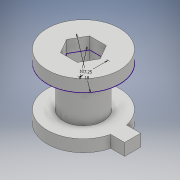
# Autodesk Inventor part: movingSpindle
Saved by Autodesk Inventor 2018 (Build 220112000, 112)
## iProperties
Created: 2018-11-25
Part Number: movingSpindle
Material: Generic
Document SubType Name: Modeling
Designer: Prakash
Density: 1 g/cm^3
Appearance: Default
Author: Prakash
Autodesk Inventor part; units mm, degrees
ref_plane "YZ Plane" through (0, 0, 0) normal (1, 0, 0) x (0, 1, 0)
ref_plane "XZ Plane" through (0, 0, 0) normal (0, 1, 0) x (-1, 0, 0)
ref_plane "XY Plane" through (0, 0, 0) normal (0, 0, 1) x (1, 0, 0)
sketch "Sketch1" plane through (0, 0, 0) normal (0, 0, 1) x (1, 0, 0)
  circle A0 centre (0, 0) radius 9
  circle A1 centre (0, 0) radius 5
  line L0 (4.1858, 0) -> (2.0929, -3.625)
  line L1 (2.0929, -3.625) -> (-2.0929, -3.625)
  line L2 (-2.0929, -3.625) -> (-4.1858, 0)
  line L3 (-4.1858, 0) -> (-2.0929, 3.625)
  line L4 (-2.0929, 3.625) -> (2.0929, 3.625)
  line L5 (2.0929, 3.625) -> (4.1858, 0)
  dimension "d1" = 18
  dimension "d2" = 10
  dimension "d3" = 7.25
  constraints: 12 end point, 3 coincident, 2 centre point, 1 horizontal, 13 other
  measures "d1" diameter of A0
  measures "d2" diameter of A1
  measures "d3" distance between parallel lines of L1 L4
extrude "Extrusion2" add sketch "Sketch1" against normal blind 10 contours A1
extrude "Extrusion4" add sketch "Sketch1" along normal blind 3 contours A0 | A1
sketch "Sketch6" plane through (0, 0, -10) normal (0, 0, -1) x (-1, 0, 0)
  circle A0 centre (0, 0) radius 9 projected
  circle A1 centre (0, 0) radius 5 projected
  line L0 (0, 0) -> (-9, 0) construction
  arc A2 (-8.775, 2) -> (-8.775, -2) centre (0, 0) ccw
  line L1 (-8.775, -2) -> (-12.275, -2)
  line L2 (-12.275, -2) -> (-12.275, 2)
  line L3 (-12.275, 2) -> (-8.775, 2)
  line L4 (-4.1858, 0) -> (-2.0929, 3.625) projected
  line L5 (-2.0929, 3.625) -> (2.0929, 3.625) projected
  line L6 (2.0929, 3.625) -> (4.1858, 0) projected
  line L7 (4.1858, 0) -> (2.0929, -3.625) projected
  line L8 (2.0929, -3.625) -> (-2.0929, -3.625) projected
  line L9 (-2.0929, -3.625) -> (-4.1858, 0) projected
  circle A3 centre (0, 0) radius 5 projected
  dimension "d20" = 3.5
  dimension "d21" = 4
  constraints: 8 end point, 6 point on circle, 2 horizontal, 2 perpendicular, 1 centre point, 1 other
  measures "d20" distance of L1.start L1.end
  measures "d21" distance between parallel lines of L3 L1
extrude "Extrusion7" add sketch "Sketch6" along normal blind 3 contours A0 | A0 L1 L2 L3 | A1
body "Solid1"
